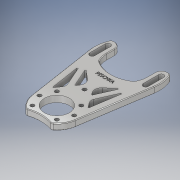
# Autodesk Inventor part: Motor Holder v3
Saved by Autodesk Inventor 2019.3 (Build 233278000, 278)
## iProperties
Created: 2019-03-01
Part Number: Motor Holder v3
Material: Aluminum 6061-AHC
Document SubType Name: Modeling
Designer: Petar
Density: 2.7 g/cm^3
Appearance: Aluminum - Dark
Mass: 26.5004 g
Surface Area: 70.5339 cm^2
Volume: 9.81495 cm^3
Author: Petar
Autodesk Inventor part; units mm, degrees
ref_plane "YZ Plane" through (0, 0, 0) normal (1, 0, 0) x (0, 1, 0)
ref_plane "XZ Plane" through (0, 0, 0) normal (0, 1, 0) x (-1, 0, 0)
ref_plane "XY Plane" through (0, 0, 0) normal (0, 0, 1) x (1, 0, 0)
sketch "Sketch1" plane through (0, 0, 0) normal (0, 1, 0) x (-1, 0, 0)
  line L0 (0, 0) -> (0, 55.6) construction
  circle A0 centre (0, 55.6) radius 10
  line L1 (16, -6.25) -> (16, 0)
  line L2 (21.213203, 18.5) -> (21.213203, -15.5) construction
  line L3 (-21.213203, 18) -> (-21.213203, -16) construction
  circle A1 centre (21.213203, 3.5) radius 1.75 construction
  circle A2 centre (21.213203, -3.5) radius 1.75 construction
  circle A3 centre (-21.213203, 3.5) radius 1.75 construction
  circle A4 centre (-21.213203, -3.5) radius 1.75 construction
  line L4 (-16, -6.25) -> (-16, 0)
  line L5 (21.213203, 6.25) -> (21.213203, -6.25) construction
  line L6 (19.213203, 6.25) -> (19.213203, -6.25)
  line L7 (23.213203, -6.25) -> (23.213203, 6.25)
  arc A5 (23.213203, 6.25) -> (19.213203, 6.25) centre (21.213203, 6.25) ccw
  arc A6 (19.213203, -6.25) -> (23.213203, -6.25) centre (21.213203, -6.25) ccw
  line L8 (-19.213203, 6.25) -> (-19.213203, -6.25)
  line L9 (-23.213203, -6.25) -> (-23.213203, 6.25)
  arc A7 (-19.213203, 6.25) -> (-23.213203, 6.25) centre (-21.213203, 6.25) ccw
  arc A8 (-23.213203, -6.25) -> (-19.213203, -6.25) centre (-21.213203, -6.25) ccw
  arc A9 (14.225426, 45.40749) -> (17.29429, 58.27536) centre (0, 55.6) ccw construction
  arc A10 (16, -6.25) -> (23.615648, -10.876635) centre (21.213203, -6.25) ccw
  arc A11 (-23.615648, -10.876635) -> (-16, -6.25) centre (-21.213203, -6.25) ccw
  line L10 (17.29429, 58.27536) -> (25.694373, 3.97482)
  line L11 (-17.29429, 58.27536) -> (-25.694373, 3.97482)
  circle A12 centre (0, 55.6) radius 13.75 construction
  circle A13 centre (9.722718, 65.322718) radius 1.5
  circle A14 centre (9.722718, 45.877282) radius 1.5
  line L12 (0, 55.6) -> (9.722718, 65.322718) construction
  line L13 (9.722718, 45.877282) -> (0, 55.6) construction
  circle A15 centre (-9.722718, 65.322718) radius 1.5
  circle A16 centre (-9.722718, 45.877282) radius 1.5
  circle A17 centre (13.75, 55.6) radius 1.5
  line L14 (13.75, 55.6) -> (0, 55.6) construction
  circle A18 centre (-13.75, 55.6) radius 1.5
  circle A19 centre (0, 33.6) radius 1.5
  line L15 (14.225426, 45.40749) -> (18.409577, 18.359942)
  arc A20 (17.29429, 58.27536) -> (-17.29429, 58.27536) centre (0, 55.6) ccw
  arc A21 (-17.29429, 58.27536) -> (-14.225426, 45.40749) centre (0, 55.6) ccw construction
  line L16 (-14.225426, 45.40749) -> (-18.409577, 18.359942)
  line L17 (10, 69.961407) -> (0, 66.6) construction
  line L18 (0, 66.6) -> (-10, 69.961407) construction
  spline S0 degree 2 poles (10, 69.961407) (0, 66.6) (-10, 69.961407) knots 1 1 1 2 2 2
  line L19 (10, 69.961407) -> (-10, 69.961407) construction
  line L20 (18.409577, 18.359942) -> (-18.409577, 18.359942) construction
  line L21 (18.409577, 18.359942) -> (10.399747, 36.52604)
  line L22 (14.225426, 45.40749) -> (10.828661, 40.666712)
  arc A22 (10.828661, 40.666712) -> (10.399747, 36.52604) centre (14.242763, 38.22051) ccw
  line L23 (-18.409577, 18.359942) -> (-10.399747, 36.52604)
  line L24 (-14.225426, 45.40749) -> (-10.828661, 40.666712)
  arc A23 (-10.399747, 36.52604) -> (-10.828661, 40.666712) centre (-14.242763, 38.22051) ccw
  line L25 (14.03801, 18.359942) -> (6.726729, 34.94175)
  line L26 (14.03801, 18.359942) -> (5.882913, 25.325705)
  line L27 (6.726729, 34.94175) -> (5.005167, 32.53901)
  arc A24 (5.005167, 32.53901) -> (5.882913, 25.325705) centre (9.371818, 29.410307) ccw
  line L28 (-14.03801, 18.359942) -> (-6.726729, 34.94175)
  line L29 (-14.03801, 18.359942) -> (-5.882913, 25.325705)
  line L30 (-6.726729, 34.94175) -> (-5.005167, 32.53901)
  arc A25 (-5.882913, 25.325705) -> (-5.005167, 32.53901) centre (-9.371818, 29.410307) ccw
  arc A26 (23.615648, -10.876635) -> (26, 0) centre (0, 0) ccw
  arc A27 (-23.615648, -10.876635) -> (23.615648, -10.876635) centre (0, 0) ccw construction
  arc A28 (-9.854282, 24.060198) -> (-25.694373, 3.97482) centre (0, 0) ccw construction
  line L31 (21.213203, -11.463203) -> (-21.213203, -11.463203) construction
  line L32 (-21.213203, 73.1) -> (25, 73.1) construction
  line L33 (0, 66.6) -> (0, 65.6) construction
  arc A29 (13.760985, 8.163043) -> (-13.760985, 8.163043) centre (0, -11.5) ccw
  line L34 (13.760985, 8.163043) -> (-13.760985, 8.163043) construction
  arc A30 (16, 0) -> (13.760985, 8.163043) centre (0, 0) ccw
  arc A31 (-13.760985, 8.163043) -> (-16, 0) centre (0, 0) ccw
  arc A32 (26, 0) -> (25.694373, 3.97482) centre (0, 0) ccw
  arc A33 (-26, 0) -> (-23.615648, -10.876635) centre (0, 0) ccw
  arc A34 (-25.694373, 3.97482) -> (-26, 0) centre (0, 0) ccw
  arc A35 (25.694373, 3.97482) -> (-11.95253, 23.08976) centre (0, 0) ccw construction
  line L35 (16, 0) -> (-16, 0) construction
  point P0 (21.213203, 0)
  point P1 (0, 12.5)
  dimension "d1" = 20
  dimension "d0" = 55.6
  dimension "d3" = 3.5
  dimension "d4" = 3.5
  dimension "d5" = 7
  dimension "d7" = 43
  dimension "d9" = 3.5
  dimension "d11" = 32
  dimension "d15" = 4
  dimension "d24" = 3
  dimension "d25" = 3
  dimension "d26" = 90
  dimension "d27" = 45
  dimension "d29" = 3
  dimension "d30" = 3
  dimension "d31" = 22
  dimension "d50" = 20
  dimension "d53" = 26
  dimension "d75" = 84.5632
  dimension "d76" = 7.5
  dimension "d77" = 3.75
  dimension "d78" = 1
  dimension "d81" = 6.25
  dimension "d82" = 12.5
  dimension "d85" = 5
  dimension "d86" = 4
  dimension "d87" = 8
  dimension "d93" = 4.2
  dimension "d98" = 15
  dimension "d99" = 24
  constraints: 70 end point, 58 point on circle, 35 centre point, 26 symmetric about line, 19 tangent, 11 point on line, 7 coincident, 5 horizontal, 5 vertical, 3 parallel, 1 collinear, 1 midpoint, 1 perpendicular, 1 vertical alignment, 16 other
  measures "d0" distance of L0.start L0.end
  measures "d3" diameter of A1
  measures "d4" diameter of A2
  measures "d5" distance of A2.centre A1.centre
  measures "d7" distance of A2.centre A3.centre
  measures "d9" vertical distance of L0.start A1.centre
  measures "d11" distance between parallel lines of L4 L1
  measures "d15" distance between parallel lines of L6 L7
  measures "d24" diameter of A13
  measures "d25" diameter of A14
  measures "d26" angle of L13 L12
  measures "d27" angle of L0 L13
  measures "d29" diameter of A17
  measures "d30" diameter of A19
  measures "d31" distance of L0.end A19.centre
  measures "d50" distance of L17.start L18.end
  measures "d53" radius of A26
  measures "d75" distance between parallel lines of L31 L32
  measures "d78" distance of L33.start L33.end
  measures "d81" vertical distance of L5.start point (0, 12.5)
  measures "d82" distance of L5.end L5.start
  measures "d85" distance between parallel lines of L10 L15
  measures "d86" distance between parallel lines of L21 L25
  measures "d93" radius of A22
  measures "d98" angle of L15 L21
  measures "d99" radius of A29
extrude "Extrusion3" add sketch "Sketch1" along normal blind 5 contours L1 A30 A29 A31 L4 A11 A33 A34 L11 A20 S0 L10 A32 A26 A10
thread "Thread1" size "M3x0.5" class "6H" standard "ANSI Metric M Profile" full length
thread "Thread2" size "M3x0.5" class "6H" standard "ANSI Metric M Profile" full length
thread "Thread3" size "M3x0.5" class "6H" standard "ANSI Metric M Profile" full length
thread "Thread4" size "M3x0.5" class "6H" standard "ANSI Metric M Profile" full length
thread "Thread5" size "M3x0.5" class "6H" standard "ANSI Metric M Profile" full length
thread "Thread6" size "M3x0.5" class "6H" standard "ANSI Metric M Profile" full length
thread "Thread7" size "M3x0.5" class "6H" standard "ANSI Metric M Profile" full length
sketch "Sketch3" plane through (0, 5, 0) normal (0, 1, 0) x (1, 0, 0)
  line L0 (-7.5, -14.6) -> (7.5, -14.6) construction
  line L1 (7.5, -14.6) -> (7.5, -19.6) construction
  line L2 (7.5, -19.6) -> (-7.5, -19.6) construction
  line L3 (-7.5, -19.6) -> (-7.5, -14.6) construction
  line L4 (0, 0) -> (0, -60) construction
  circle A0 centre (0, -33.6) radius 1.5
  spline S0 degree 2 poles (-5.043979, -16.595705) (-5.043979, -16.760373) (-5.161305, -17.056775) (-5.266281, -17.159692) knots 0 0 0 1 2 2 2
  spline S1 degree 2 poles (-5.266281, -17.159692) (-5.398015, -17.289368) (-5.754109, -17.423161) (-6.025811, -17.423161) knots 0 0 0 1 2 2 2
  line L5 (-6.025811, -17.423161) -> (-6.311921, -17.423161)
  line L6 (-6.311921, -17.423161) -> (-6.311921, -18.37)
  line L7 (-6.311921, -18.37) -> (-6.64949, -18.37)
  line L8 (-6.64949, -18.37) -> (-6.64949, -15.83)
  line L9 (-6.64949, -15.83) -> (-6.011402, -15.83)
  spline S2 degree 2 poles (-6.011402, -15.83) (-5.784984, -15.83) (-5.467998, -15.9041) (-5.346556, -15.988493) knots 0 0 0 1 2 2 2
  spline S3 degree 2 poles (-5.346556, -15.988493) (-5.20453, -16.085235) (-5.043979, -16.383695) (-5.043979, -16.595705) knots 0 0 0 1 2 2 2
  spline S4 degree 2 poles (-5.395956, -16.605997) (-5.395956, -16.474263) (-5.486524, -16.280778) (-5.579149, -16.219028) knots 0 0 0 1 2 2 2
  spline S5 degree 2 poles (-5.579149, -16.219028) (-5.659425, -16.165511) (-5.873493, -16.122285) (-6.031986, -16.122285) knots 0 0 0 1 2 2 2
  line L10 (-6.031986, -16.122285) -> (-6.311921, -16.122285)
  line L11 (-6.311921, -16.122285) -> (-6.311921, -17.134992)
  line L12 (-6.311921, -17.134992) -> (-6.081386, -17.134992)
  spline S6 degree 2 poles (-6.081386, -17.134992) (-5.875551, -17.134992) (-5.622375, -17.069125) (-5.540041, -16.982674) knots 0 0 0 1 2 2 2
  spline S7 degree 2 poles (-5.540041, -16.982674) (-5.463882, -16.906515) (-5.395956, -16.727439) (-5.395956, -16.605997) knots 0 0 0 1 2 2 2
  line L13 (-3.837788, -18.37) -> (-4.821678, -18.37)
  line L14 (-4.821678, -18.37) -> (-4.821678, -18.110648)
  line L15 (-4.821678, -18.110648) -> (-4.498517, -18.110648)
  line L16 (-4.498517, -18.110648) -> (-4.498517, -16.089352)
  line L17 (-4.498517, -16.089352) -> (-4.821678, -16.089352)
  line L18 (-4.821678, -16.089352) -> (-4.821678, -15.83)
  line L19 (-4.821678, -15.83) -> (-3.837788, -15.83)
  line L20 (-3.837788, -15.83) -> (-3.837788, -16.089352)
  line L21 (-3.837788, -16.089352) -> (-4.160948, -16.089352)
  line L22 (-4.160948, -16.089352) -> (-4.160948, -18.110648)
  line L23 (-4.160948, -18.110648) -> (-3.837788, -18.110648)
  line L24 (-3.837788, -18.110648) -> (-3.837788, -18.37)
  spline S8 degree 2 poles (-2.711872, -18.415284) (-2.98769, -18.415284) (-3.37466, -18.300016) (-3.545502, -18.217682) knots 0 0 0 1 2 2 2
  line L25 (-3.545502, -18.217682) -> (-3.545502, -17.793663)
  line L26 (-3.545502, -17.793663) -> (-3.520802, -17.793663)
  spline S9 degree 2 poles (-3.520802, -17.793663) (-3.354076, -17.950097) (-2.932115, -18.122998) (-2.736572, -18.122998) knots 0 0 0 1 2 2 2
  spline S10 degree 2 poles (-2.736572, -18.122998) (-2.456637, -18.122998) (-2.170527, -17.890405) (-2.170527, -17.698979) knots 0 0 0 1 2 2 2
  spline S11 degree 2 poles (-2.170527, -17.698979) (-2.170527, -17.546661) (-2.320786, -17.357293) (-2.483395, -17.309951) knots 0 0 0 1 2 2 2
  spline S12 degree 2 poles (-2.483395, -17.309951) (-2.600721, -17.277018) (-2.796264, -17.231734) (-2.942407, -17.194684) knots 0 0 0 1 2 2 2
  spline S13 degree 2 poles (-2.942407, -17.194684) (-3.074141, -17.159692) (-3.282034, -17.054716) (-3.36231, -16.970324) knots 0 0 0 1 2 2 2
  spline S14 degree 2 poles (-3.36231, -16.970324) (-3.440527, -16.885932) (-3.526977, -16.659514) (-3.526977, -16.511313) knots 0 0 0 1 2 2 2
  spline S15 degree 2 poles (-3.526977, -16.511313) (-3.526977, -16.202561) (-3.045324, -15.784716) (-2.672763, -15.784716) knots 0 0 0 1 2 2 2
  spline S16 degree 2 poles (-2.672763, -15.784716) (-2.458695, -15.784716) (-2.079959, -15.869109) (-1.91735, -15.949384) knots 0 0 0 1 2 2 2
  line L27 (-1.91735, -15.949384) -> (-1.91735, -16.35282)
  line L28 (-1.91735, -16.35282) -> (-1.94205, -16.35282)
  spline S17 degree 2 poles (-1.94205, -16.35282) (-2.063493, -16.241669) (-2.442229, -16.077002) (-2.650122, -16.077002) knots 0 0 0 1 2 2 2
  spline S18 degree 2 poles (-2.650122, -16.077002) (-2.884773, -16.077002) (-3.175, -16.297245) (-3.175, -16.476321) knots 0 0 0 1 2 2 2
  spline S19 degree 2 poles (-3.175, -16.476321) (-3.175, -16.636872) (-3.004157, -16.828298) (-2.843606, -16.871524) knots 0 0 0 1 2 2 2
  spline S20 degree 2 poles (-2.843606, -16.871524) (-2.736572, -16.90034) (-2.425762, -16.974441) (-2.322844, -17.005316) knots 0 0 0 1 2 2 2
  spline S21 degree 2 poles (-2.322844, -17.005316) (-2.061434, -17.085592) (-1.818549, -17.408752) (-1.818549, -17.645462) knots 0 0 0 1 2 2 2
  spline S22 degree 2 poles (-1.818549, -17.645462) (-1.818549, -17.795721) (-1.939992, -18.08389) (-2.049084, -18.184749) knots 0 0 0 1 2 2 2
  spline S23 degree 2 poles (-2.049084, -18.184749) (-2.170527, -18.2959) (-2.479279, -18.415284) (-2.711872, -18.415284) knots 0 0 0 1 2 2 2
  spline S24 degree 2 poles (-0.482682, -18.415284) (-0.729684, -18.415284) (-1.147528, -18.248558) (-1.299846, -18.081832) knots 0 0 0 1 2 2 2
  spline S25 degree 2 poles (-1.299846, -18.081832) (-1.452164, -17.917164) (-1.61889, -17.423161) (-1.61889, -17.102058) knots 0 0 0 1 2 2 2
  spline S26 degree 2 poles (-1.61889, -17.102058) (-1.61889, -16.783015) (-1.45628, -16.309595) (-1.301904, -16.134635) knots 0 0 0 1 2 2 2
  spline S27 degree 2 poles (-1.301904, -16.134635) (-1.149587, -15.963793) (-0.733801, -15.784716) (-0.476507, -15.784716) knots 0 0 0 1 2 2 2
  spline S28 degree 2 poles (-0.476507, -15.784716) (-0.34889, -15.784716) (-0.12453, -15.821767) (-0.029846, -15.850583) knots 0 0 0 1 2 2 2
  spline S29 degree 2 poles (-0.029846, -15.850583) (0.052488, -15.877342) (0.223331, -15.953501) (0.307723, -15.998784) knots 0 0 0 1 2 2 2
  line L29 (0.307723, -15.998784) -> (0.307723, -16.406337)
  line L30 (0.307723, -16.406337) -> (0.280964, -16.406337)
  spline S30 degree 2 poles (0.280964, -16.406337) (0.235681, -16.36517) (0.095713, -16.249903) (-0.005146, -16.194327) knots 0 0 0 1 2 2 2
  spline S31 degree 2 poles (-0.005146, -16.194327) (-0.101888, -16.14081) (-0.330365, -16.072885) (-0.478566, -16.072885) knots 0 0 0 1 2 2 2
  spline S32 degree 2 poles (-0.478566, -16.072885) (-0.641175, -16.072885) (-0.931402, -16.206677) (-1.040494, -16.334295) knots 0 0 0 1 2 2 2
  spline S33 degree 2 poles (-1.040494, -16.334295) (-1.147528, -16.463971) (-1.266912, -16.857115) (-1.266912, -17.102058) knots 0 0 0 1 2 2 2
  spline S34 degree 2 poles (-1.266912, -17.102058) (-1.266912, -17.363468) (-1.141353, -17.740146) (-1.032261, -17.869822) knots 0 0 0 1 2 2 2
  spline S35 degree 2 poles (-1.032261, -17.869822) (-0.925227, -17.995381) (-0.639117, -18.122998) (-0.478566, -18.122998) knots 0 0 0 1 2 2 2
  spline S36 degree 2 poles (-0.478566, -18.122998) (-0.332423, -18.122998) (-0.083363, -18.050956) (0.013379, -17.997439) knots 0 0 0 1 2 2 2
  spline S37 degree 2 poles (0.013379, -17.997439) (0.106005, -17.943922) (0.243914, -17.832772) (0.283023, -17.793663) knots 0 0 0 1 2 2 2
  line L31 (0.283023, -17.793663) -> (0.307723, -17.793663)
  line L32 (0.307723, -17.793663) -> (0.307723, -18.197099)
  spline S38 degree 2 poles (0.307723, -18.197099) (0.223331, -18.236208) (0.07513, -18.30825) (-0.029846, -18.341183) knots 0 0 0 1 2 2 2
  spline S39 degree 2 poles (-0.029846, -18.341183) (-0.140997, -18.378233) (-0.330365, -18.415284) (-0.482682, -18.415284) knots 0 0 0 1 2 2 2
  line L33 (2.466929, -18.37) -> (2.12936, -18.37)
  line L34 (2.12936, -18.37) -> (2.12936, -17.126759)
  line L35 (2.12936, -17.126759) -> (0.960219, -17.126759)
  line L36 (0.960219, -17.126759) -> (0.960219, -18.37)
  line L37 (0.960219, -18.37) -> (0.62265, -18.37)
  line L38 (0.62265, -18.37) -> (0.62265, -15.83)
  line L39 (0.62265, -15.83) -> (0.960219, -15.83)
  line L40 (0.960219, -15.83) -> (0.960219, -16.82624)
  line L41 (0.960219, -16.82624) -> (2.12936, -16.82624)
  line L42 (2.12936, -16.82624) -> (2.12936, -15.83)
  line L43 (2.12936, -15.83) -> (2.466929, -15.83)
  line L44 (2.466929, -15.83) -> (2.466929, -18.37)
  line L45 (4.834028, -18.37) -> (4.3956, -18.37)
  line L46 (4.3956, -18.37) -> (3.467285, -17.188509)
  line L47 (3.467285, -17.188509) -> (3.319084, -17.355235)
  line L48 (3.319084, -17.355235) -> (3.319084, -18.37)
  line L49 (3.319084, -18.37) -> (2.981516, -18.37)
  line L50 (2.981516, -18.37) -> (2.981516, -15.83)
  line L51 (2.981516, -15.83) -> (3.319084, -15.83)
  line L52 (3.319084, -15.83) -> (3.319084, -16.997083)
  line L53 (3.319084, -16.997083) -> (4.360608, -15.83)
  line L54 (4.360608, -15.83) -> (4.772277, -15.83)
  line L55 (4.772277, -15.83) -> (3.720462, -16.964149)
  line L56 (3.720462, -16.964149) -> (4.834028, -18.37)
  line L57 (4.761986, -18.37) -> (5.618258, -15.83)
  line L58 (5.618258, -15.83) -> (6.034044, -15.83)
  line L59 (6.034044, -15.83) -> (6.890316, -18.37)
  line L60 (6.890316, -18.37) -> (6.534222, -18.37)
  line L61 (6.534222, -18.37) -> (6.303687, -17.65987)
  line L62 (6.303687, -17.65987) -> (5.334206, -17.65987)
  line L63 (5.334206, -17.65987) -> (5.103671, -18.37)
  line L64 (5.103671, -18.37) -> (4.761986, -18.37)
  line L65 (6.211062, -17.371702) -> (5.817918, -16.175802)
  line L66 (5.817918, -16.175802) -> (5.426832, -17.371702)
  line L67 (5.426832, -17.371702) -> (6.211062, -17.371702)
  dimension "d68" = 14
  dimension "d69" = 5
  dimension "d70" = 15
  constraints: 2 end point, 1 vertical, 3 other
  measures "d68" distance from line of L2 A0.centre
  measures "d69" distance between parallel lines of L0 L2
  measures "d70" distance between parallel lines of L3 L1
emboss "Emboss1" sketch "Sketch3" operation cut depth 0.2 direction (0, -1, 0) contours S0 S1 L5 L6 L7 L8 L9 S2 S3 | L13 L14 L15 L16 L17 L18 L19 L20 L21 L22 L23 L24 | S8 L25 L26 S9 S10 S11 S12 S13 S14 S15 S16 L27 L28 S17 S18 S19 S20 S21 S22 S23 | S24 S25 S26 S27 S28 S29 L29 L30 S30 S31 S32 S33 S34 S35 S36 S37 L31 L32 S38 S39 | L33 L34 L35 L36 L37 L38 L39 L40 L41 L42 L43 L44 | L45 L57 L56 | L56 L57 L58 L59 L60 L61 L62 L63 L64 | L45 L46 L47 L48 L49 L50 L51 L52 L53 L54 L55 L56 L57
sketch "Sketch4" plane through (0, 0, 0) normal (0, -1, 0) x (1, 0, 0)
  circle A0 centre (0, 33.6) radius 1.5
  line L0 (7.5, 14.6) -> (-7.5, 14.6) construction
  line L1 (-7.5, 14.6) -> (-7.5, 19.6) construction
  line L2 (-7.5, 19.6) -> (7.5, 19.6) construction
  line L3 (7.5, 19.6) -> (7.5, 14.6) construction
  spline S0 degree 2 poles (5.043979, 16.595705) (5.043979, 16.760373) (5.161305, 17.056775) (5.266281, 17.159692) knots 0 0 0 1 2 2 2
  spline S1 degree 2 poles (5.266281, 17.159692) (5.398015, 17.289368) (5.754109, 17.423161) (6.025811, 17.423161) knots 0 0 0 1 2 2 2
  line L4 (6.025811, 17.423161) -> (6.311921, 17.423161)
  line L5 (6.311921, 17.423161) -> (6.311921, 18.37)
  line L6 (6.311921, 18.37) -> (6.64949, 18.37)
  line L7 (6.64949, 18.37) -> (6.64949, 15.83)
  line L8 (6.64949, 15.83) -> (6.011402, 15.83)
  spline S2 degree 2 poles (6.011402, 15.83) (5.784984, 15.83) (5.467998, 15.9041) (5.346556, 15.988493) knots 0 0 0 1 2 2 2
  spline S3 degree 2 poles (5.346556, 15.988493) (5.20453, 16.085235) (5.043979, 16.383695) (5.043979, 16.595705) knots 0 0 0 1 2 2 2
  spline S4 degree 2 poles (5.395956, 16.605997) (5.395956, 16.474263) (5.486524, 16.280778) (5.579149, 16.219028) knots 0 0 0 1 2 2 2
  spline S5 degree 2 poles (5.579149, 16.219028) (5.659425, 16.165511) (5.873493, 16.122285) (6.031986, 16.122285) knots 0 0 0 1 2 2 2
  line L9 (6.031986, 16.122285) -> (6.311921, 16.122285)
  line L10 (6.311921, 16.122285) -> (6.311921, 17.134992)
  line L11 (6.311921, 17.134992) -> (6.081386, 17.134992)
  spline S6 degree 2 poles (6.081386, 17.134992) (5.875551, 17.134992) (5.622375, 17.069125) (5.540041, 16.982674) knots 0 0 0 1 2 2 2
  spline S7 degree 2 poles (5.540041, 16.982674) (5.463882, 16.906515) (5.395956, 16.727439) (5.395956, 16.605997) knots 0 0 0 1 2 2 2
  line L12 (3.837788, 18.37) -> (4.821678, 18.37)
  line L13 (4.821678, 18.37) -> (4.821678, 18.110648)
  line L14 (4.821678, 18.110648) -> (4.498517, 18.110648)
  line L15 (4.498517, 18.110648) -> (4.498517, 16.089352)
  line L16 (4.498517, 16.089352) -> (4.821678, 16.089352)
  line L17 (4.821678, 16.089352) -> (4.821678, 15.83)
  line L18 (4.821678, 15.83) -> (3.837788, 15.83)
  line L19 (3.837788, 15.83) -> (3.837788, 16.089352)
  line L20 (3.837788, 16.089352) -> (4.160948, 16.089352)
  line L21 (4.160948, 16.089352) -> (4.160948, 18.110648)
  line L22 (4.160948, 18.110648) -> (3.837788, 18.110648)
  line L23 (3.837788, 18.110648) -> (3.837788, 18.37)
  spline S8 degree 2 poles (2.711872, 18.415284) (2.98769, 18.415284) (3.37466, 18.300016) (3.545502, 18.217682) knots 0 0 0 1 2 2 2
  line L24 (3.545502, 18.217682) -> (3.545502, 17.793663)
  line L25 (3.545502, 17.793663) -> (3.520802, 17.793663)
  spline S9 degree 2 poles (3.520802, 17.793663) (3.354076, 17.950097) (2.932115, 18.122998) (2.736572, 18.122998) knots 0 0 0 1 2 2 2
  spline S10 degree 2 poles (2.736572, 18.122998) (2.456637, 18.122998) (2.170527, 17.890405) (2.170527, 17.698979) knots 0 0 0 1 2 2 2
  spline S11 degree 2 poles (2.170527, 17.698979) (2.170527, 17.546661) (2.320786, 17.357293) (2.483395, 17.309951) knots 0 0 0 1 2 2 2
  spline S12 degree 2 poles (2.483395, 17.309951) (2.600721, 17.277018) (2.796264, 17.231734) (2.942407, 17.194684) knots 0 0 0 1 2 2 2
  spline S13 degree 2 poles (2.942407, 17.194684) (3.074141, 17.159692) (3.282034, 17.054716) (3.36231, 16.970324) knots 0 0 0 1 2 2 2
  spline S14 degree 2 poles (3.36231, 16.970324) (3.440527, 16.885932) (3.526977, 16.659514) (3.526977, 16.511313) knots 0 0 0 1 2 2 2
  spline S15 degree 2 poles (3.526977, 16.511313) (3.526977, 16.202561) (3.045324, 15.784716) (2.672763, 15.784716) knots 0 0 0 1 2 2 2
  spline S16 degree 2 poles (2.672763, 15.784716) (2.458695, 15.784716) (2.079959, 15.869109) (1.91735, 15.949384) knots 0 0 0 1 2 2 2
  line L26 (1.91735, 15.949384) -> (1.91735, 16.35282)
  line L27 (1.91735, 16.35282) -> (1.94205, 16.35282)
  spline S17 degree 2 poles (1.94205, 16.35282) (2.063493, 16.241669) (2.442229, 16.077002) (2.650122, 16.077002) knots 0 0 0 1 2 2 2
  spline S18 degree 2 poles (2.650122, 16.077002) (2.884773, 16.077002) (3.175, 16.297245) (3.175, 16.476321) knots 0 0 0 1 2 2 2
  spline S19 degree 2 poles (3.175, 16.476321) (3.175, 16.636872) (3.004157, 16.828298) (2.843606, 16.871524) knots 0 0 0 1 2 2 2
  spline S20 degree 2 poles (2.843606, 16.871524) (2.736572, 16.90034) (2.425762, 16.974441) (2.322844, 17.005316) knots 0 0 0 1 2 2 2
  spline S21 degree 2 poles (2.322844, 17.005316) (2.061434, 17.085592) (1.818549, 17.408752) (1.818549, 17.645462) knots 0 0 0 1 2 2 2
  spline S22 degree 2 poles (1.818549, 17.645462) (1.818549, 17.795721) (1.939992, 18.08389) (2.049084, 18.184749) knots 0 0 0 1 2 2 2
  spline S23 degree 2 poles (2.049084, 18.184749) (2.170527, 18.2959) (2.479279, 18.415284) (2.711872, 18.415284) knots 0 0 0 1 2 2 2
  spline S24 degree 2 poles (0.482682, 18.415284) (0.729684, 18.415284) (1.147528, 18.248558) (1.299846, 18.081832) knots 0 0 0 1 2 2 2
  spline S25 degree 2 poles (1.299846, 18.081832) (1.452164, 17.917164) (1.61889, 17.423161) (1.61889, 17.102058) knots 0 0 0 1 2 2 2
  spline S26 degree 2 poles (1.61889, 17.102058) (1.61889, 16.783015) (1.45628, 16.309595) (1.301904, 16.134635) knots 0 0 0 1 2 2 2
  spline S27 degree 2 poles (1.301904, 16.134635) (1.149587, 15.963793) (0.733801, 15.784716) (0.476507, 15.784716) knots 0 0 0 1 2 2 2
  spline S28 degree 2 poles (0.476507, 15.784716) (0.34889, 15.784716) (0.12453, 15.821767) (0.029846, 15.850583) knots 0 0 0 1 2 2 2
  spline S29 degree 2 poles (0.029846, 15.850583) (-0.052488, 15.877342) (-0.223331, 15.953501) (-0.307723, 15.998784) knots 0 0 0 1 2 2 2
  line L28 (-0.307723, 15.998784) -> (-0.307723, 16.406337)
  line L29 (-0.307723, 16.406337) -> (-0.280964, 16.406337)
  spline S30 degree 2 poles (-0.280964, 16.406337) (-0.235681, 16.36517) (-0.095713, 16.249903) (0.005146, 16.194327) knots 0 0 0 1 2 2 2
  spline S31 degree 2 poles (0.005146, 16.194327) (0.101888, 16.14081) (0.330365, 16.072885) (0.478566, 16.072885) knots 0 0 0 1 2 2 2
  spline S32 degree 2 poles (0.478566, 16.072885) (0.641175, 16.072885) (0.931402, 16.206677) (1.040494, 16.334295) knots 0 0 0 1 2 2 2
  spline S33 degree 2 poles (1.040494, 16.334295) (1.147528, 16.463971) (1.266912, 16.857115) (1.266912, 17.102058) knots 0 0 0 1 2 2 2
  spline S34 degree 2 poles (1.266912, 17.102058) (1.266912, 17.363468) (1.141353, 17.740146) (1.032261, 17.869822) knots 0 0 0 1 2 2 2
  spline S35 degree 2 poles (1.032261, 17.869822) (0.925227, 17.995381) (0.639117, 18.122998) (0.478566, 18.122998) knots 0 0 0 1 2 2 2
  spline S36 degree 2 poles (0.478566, 18.122998) (0.332423, 18.122998) (0.083363, 18.050956) (-0.013379, 17.997439) knots 0 0 0 1 2 2 2
  spline S37 degree 2 poles (-0.013379, 17.997439) (-0.106005, 17.943922) (-0.243914, 17.832772) (-0.283023, 17.793663) knots 0 0 0 1 2 2 2
  line L30 (-0.283023, 17.793663) -> (-0.307723, 17.793663)
  line L31 (-0.307723, 17.793663) -> (-0.307723, 18.197099)
  spline S38 degree 2 poles (-0.307723, 18.197099) (-0.223331, 18.236208) (-0.07513, 18.30825) (0.029846, 18.341183) knots 0 0 0 1 2 2 2
  spline S39 degree 2 poles (0.029846, 18.341183) (0.140997, 18.378233) (0.330365, 18.415284) (0.482682, 18.415284) knots 0 0 0 1 2 2 2
  line L32 (-2.466929, 18.37) -> (-2.12936, 18.37)
  line L33 (-2.12936, 18.37) -> (-2.12936, 17.126759)
  line L34 (-2.12936, 17.126759) -> (-0.960219, 17.126759)
  line L35 (-0.960219, 17.126759) -> (-0.960219, 18.37)
  line L36 (-0.960219, 18.37) -> (-0.62265, 18.37)
  line L37 (-0.62265, 18.37) -> (-0.62265, 15.83)
  line L38 (-0.62265, 15.83) -> (-0.960219, 15.83)
  line L39 (-0.960219, 15.83) -> (-0.960219, 16.82624)
  line L40 (-0.960219, 16.82624) -> (-2.12936, 16.82624)
  line L41 (-2.12936, 16.82624) -> (-2.12936, 15.83)
  line L42 (-2.12936, 15.83) -> (-2.466929, 15.83)
  line L43 (-2.466929, 15.83) -> (-2.466929, 18.37)
  line L44 (-4.834028, 18.37) -> (-4.3956, 18.37)
  line L45 (-4.3956, 18.37) -> (-3.467285, 17.188509)
  line L46 (-3.467285, 17.188509) -> (-3.319084, 17.355235)
  line L47 (-3.319084, 17.355235) -> (-3.319084, 18.37)
  line L48 (-3.319084, 18.37) -> (-2.981516, 18.37)
  line L49 (-2.981516, 18.37) -> (-2.981516, 15.83)
  line L50 (-2.981516, 15.83) -> (-3.319084, 15.83)
  line L51 (-3.319084, 15.83) -> (-3.319084, 16.997083)
  line L52 (-3.319084, 16.997083) -> (-4.360608, 15.83)
  line L53 (-4.360608, 15.83) -> (-4.772277, 15.83)
  line L54 (-4.772277, 15.83) -> (-3.720462, 16.964149)
  line L55 (-3.720462, 16.964149) -> (-4.834028, 18.37)
  line L56 (-4.761986, 18.37) -> (-5.618258, 15.83)
  line L57 (-5.618258, 15.83) -> (-6.034044, 15.83)
  line L58 (-6.034044, 15.83) -> (-6.890316, 18.37)
  line L59 (-6.890316, 18.37) -> (-6.534222, 18.37)
  line L60 (-6.534222, 18.37) -> (-6.303687, 17.65987)
  line L61 (-6.303687, 17.65987) -> (-5.334206, 17.65987)
  line L62 (-5.334206, 17.65987) -> (-5.103671, 18.37)
  line L63 (-5.103671, 18.37) -> (-4.761986, 18.37)
  line L64 (-6.211062, 17.371702) -> (-5.817918, 16.175802)
  line L65 (-5.817918, 16.175802) -> (-5.426832, 17.371702)
  line L66 (-5.426832, 17.371702) -> (-6.211062, 17.371702)
  dimension "d67" = 14
  dimension "d71" = 5
  dimension "d72" = 15
  constraints: 2 other
  measures "d67" distance from line of L2 A0.centre
  measures "d71" distance between parallel lines of L2 L0
  measures "d72" distance between parallel lines of L3 L1
emboss "Emboss2" sketch "Sketch4" operation cut depth 0.2 direction (0, 1, 0) contours S0 S1 L4 L5 L6 L7 L8 S2 S3 | L12 L13 L14 L15 L16 L17 L18 L19 L20 L21 L22 L23 | S8 L24 L25 S9 S10 S11 S12 S13 S14 S15 S16 L26 L27 S17 S18 S19 S20 S21 S22 S23 | S24 S25 S26 S27 S28 S29 L28 L29 S30 S31 S32 S33 S34 S35 S36 S37 L30 L31 S38 S39 | L32 L33 L34 L35 L36 L37 L38 L39 L40 L41 L42 L43 | L44 L56 L55 | L55 L56 L57 L58 L59 L60 L61 L62 L63 | L44 L45 L46 L47 L48 L49 L50 L51 L52 L53 L54 L55 L56
fillet "Fillet3" radius 0.5 8 edges at (-18.4096, 2.5, 18.3599) (-14.038, 2.5, 18.3599) (-6.7267, 2.5, 34.9418) (-14.2254, 2.5, 45.4075) (6.7267, 2.5, 34.9418) (14.2254, 2.5, 45.4075) (18.4096, 2.5, 18.3599) (14.038, 2.5, 18.3599)
fillet "Fillet5" radius 2 6 edges at (-10, 2.5, 69.9614) (10, 2.5, 69.9614) (23.6156, 2.5, -10.8766) (-23.6156, 2.5, -10.8766) (-13.761, 2.5, 8.163) (13.761, 2.5, 8.163)
chamfer "Chamfer3" distance 0.5 angle 45 40 edges at (15.1269, 5, 64.3993) (21.4943, 5, 31.1251) (10.0052, 5, 69.7087) (0, 5, 68.2807) (-10.0052, 5, 69.7087) (-15.1269, 5, 64.3993) (-21.4943, 5, 31.1251) (-25.8035, 5, -3.1905) (-23.4392, 5, -10.8298) (-18.0833, 5, -10.419) (-16, 5, -3.125) (-15.4929, 5, 3.9962) (-13.7269, 5, 8.124) (0, 5, 12.5) (13.7269, 5, 8.124) (15.4929, 5, 3.9962) (16, 5, -3.125) (18.0833, 5, -10.419) (23.4392, 5, -10.8298) (25.8035, 5, -3.1905) (0, 0, 68.2807) (10.0052, 0, 69.7087) (15.1269, 0, 64.3993) (21.4943, 0, 31.1251) (-10.0052, 0, 69.7087) (-15.1269, 0, 64.3993) (-21.4943, 0, 31.1251) (-25.8035, 0, -3.1905) (-23.4392, 0, -10.8298) (-18.0833, 0, -10.419) (-16, 0, -3.125) (-15.4929, 0, 3.9962) (-13.7269, 0, 8.124) (0, 0, 12.5) (13.7269, 0, 8.124) (15.4929, 0, 3.9962) (16, 0, -3.125) (18.0833, 0, -10.419) (23.4392, 0, -10.8298) (25.8035, 0, -3.1905)
sketch "Center Lines" plane through (0, 5, 0) normal (0, 1, 0) x (1, 0, 0)
  arc A0 (-23.213203, -6.25) -> (-19.213203, -6.25) centre (-21.213203, -6.25) ccw construction
  line L0 (-23.213203, -6.25) -> (-23.213203, 6.25) construction
  arc A1 (-19.213203, 6.25) -> (-23.213203, 6.25) centre (-21.213203, 6.25) ccw construction
  line L1 (-19.213203, 6.25) -> (-19.213203, -6.25) construction
  line L2 (-21.213203, -6.25) -> (-21.213203, 6.25) construction
  line L3 (19.213203, -6.25) -> (19.213203, 6.25) construction
  arc A2 (19.213203, -6.25) -> (23.213203, -6.25) centre (21.213203, -6.25) ccw construction
  line L4 (23.213203, 6.25) -> (23.213203, -6.25) construction
  arc A3 (23.213203, 6.25) -> (19.213203, 6.25) centre (21.213203, 6.25) ccw construction
  line L5 (21.213203, -6.25) -> (21.213203, 6.25) construction
  constraints: 4 end point, 2 vertical
body "Solid3"
